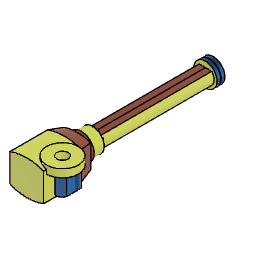
Jaw_3 v3 (Autodesk Fusion 360 design; units mm, degrees)
Autodesk Fusion 360 part; units mm, degrees
sketch "Sketch1" plane through (0, 0, 0) normal (0, 1, 0) x (1, 0, 0)
  line L0 (0, 0) -> (0, 45)
  line L1 (0, 0) -> (0, -45)
  line L2 (0, 45) -> (37.5, 45)
  line L3 (0, 45) -> (-37.5, 45)
  line L4 (0, -45) -> (37.5, -45)
  line L5 (0, -45) -> (-37.5, -45)
  arc A0 (-37.5, 45) -> (-37.5, -45) centre (79.119, 0) ccw
  arc A1 (37.5, -45) -> (37.5, 45) centre (-79.119, 0) ccw
  dimension "d1" = 45
  dimension "d2" = 45
  dimension "d3" = 37.5
  dimension "d4" = 37.5
  dimension "d5" = 37.5
  dimension "d6" = 37.5
  dimension "d7" = 125
  dimension "d8" = 125
  constraint coincident L0.start L1.start
  measures "d1" distance of L0.start L0.end
  measures "d2" distance of L0.start L1.end
  measures "d3" distance of L0.end L2.end
  measures "d4" distance of L0.end L3.end
  measures "d5" distance of L1.end L4.end
  measures "d6" distance of L1.end L5.end
  measures "d7" radius of A0
  measures "d8" radius of A1
sketch "Sketch2" plane through (0, 145, 0) normal (0, 1, 0) x (-1, 0, 0)
  circle A0 centre (0, 0) radius 34.5
  circle A1 centre (0, 0) radius 31
  dimension "d9" = 62
  constraint concentric A0 A1
  measures "d9" diameter of A1
sketch "Sketch3" plane through (0, 135, 0) normal (0, 1, 0) x (-1, 0, 0)
  line L0 (30.8786, 35.6218) -> (-30.8786, 35.6218)
  arc A0 (-30.8786, 35.6218) -> (-30.8786, -35.6218) centre (79.119, 0) ccw
  line L1 (-30.8786, -35.6218) -> (30.8786, -35.6218)
  arc A1 (30.8786, -35.6218) -> (30.8786, 35.6218) centre (-79.119, 0) ccw
  circle A2 centre (0, 0) radius 34.5
  dimension "d10" = 69
  constraint coincident A2.centre origin
  measures "d10" diameter of A2
sketch "Sketch4" plane through (0, 175, 0) normal (0, 1, 0) x (-1, 0, 0)
  circle A0 centre (0, 0) radius 31
  line L0 (0, 0) -> (-27, 0)
  circle A1 centre (-27, 0) radius 2.5
  circle A2 centre (-27, 0) radius 3.5
  dimension "d11" = 27
  dimension "d12" = 5
  dimension "d13" = 1
  constraint coincident A0.centre L0.start
  constraint coincident L0.end A1.centre
  measures "d11" distance of A0.centre L0.end
  measures "d12" diameter of A1
sketch "Sketch5" plane through (0, 175, 0) normal (0, 1, 0) x (-1, 0, 0)
  circle A0 centre (-13.5, 23.3827) radius 3.5
  circle A1 centre (13.5, 23.3827) radius 3.5
  circle A2 centre (27, 0) radius 3.5
  circle A3 centre (13.5, -23.3827) radius 3.5
  circle A4 centre (-13.5, -23.3827) radius 3.5
  circle A5 centre (-27, 0) radius 3.5
  circle A6 centre (0, 0) radius 31
  circle A7 centre (-23.3827, -13.5) radius 3.5
  circle A8 centre (0, -27) radius 3.5
  circle A9 centre (23.3827, -13.5) radius 3.5
  circle A10 centre (23.3827, 13.5) radius 3.5
  circle A11 centre (0, 27) radius 3.5
  circle A12 centre (-23.3827, 13.5) radius 3.5
  line L0 (-15.9819, 0.0787) -> (-15.9461, -16.9213)
  line L1 (-15.9819, 0.0787) -> (-15.9602, 17.0787)
  line L2 (16, 0) -> (16.0134, -16.8465)
  line L3 (16, 0) -> (16, 17)
  arc A13 (-15.9461, -16.9213) -> (16.0134, -16.8465) centre (-0.0069, 0.4409) ccw
  arc A14 (16, 17) -> (-15.9602, 17.0787) centre (-0.0232, -0.4651) ccw
  dimension "d14" = 17
  dimension "d15" = 17
  dimension "d16" = 23.5691
  measures "d14" distance of L0.start L0.end
  measures "d15" distance of L0.start L1.end
  measures "d16" radius of A13
sketch "Sketch6" plane through (0, 275, 0) normal (0, 1, 0) x (-1, 0, 0)
  line L0 (16, 0) -> (16, 17)
  arc A0 (16, 17) -> (-15.9602, 17.0787) centre (-0.0232, -0.4651) ccw
  line L1 (-15.9602, 17.0787) -> (-15.9819, 0.0787)
  line L2 (-15.9819, 0.0787) -> (-15.9461, -16.9213)
  arc A1 (-15.9461, -16.9213) -> (16.0134, -16.8465) centre (-0.0069, 0.4409) ccw
  line L3 (16.0134, -16.8465) -> (16, 0)
  circle A2 centre (0, 0) radius 31
  point P0 (-31, 0)
  constraint coincident A2.centre origin
  constraint coincident A2 P0
sketch "Sketch7" plane through (0, 285, 0) normal (0, 1, 0) x (-1, 0, 0)
  circle A0 centre (0, 0) radius 31
  circle A1 centre (0, 0) radius 30
  dimension "d17" = 1
sketch "Sketch8" plane through (-37.5, 0, -45) normal (-1, 0, 0) x (0, 0, -1)
  circle A0 centre (-90, -50) radius 42.5
  line L0 (-90, 0) -> (-90, -100)
  dimension "d18" = 85
  constraint midpoint A0.centre L0
  measures "d18" diameter of A0
sketch "Sketch9" plane through (0, 286, 0) normal (0, 1, 0) x (-1, 0, 0)
  circle A0 centre (0, 0) radius 30
  circle A1 centre (0, 0) radius 31
  circle A2 centre (0, 0) radius 31
  circle A3 centre (0, 0) radius 31
  constraint coincident A0.centre A1.centre
sketch "Sketch10" plane through (-48, 0, 0) normal (-1, 0, 0) x (0, 0, 1)
  circle A0 centre (45, 50) radius 42.5
  circle A1 centre (45, 50) radius 15
  dimension "d19" = 30
  constraint concentric A0 A1
  measures "d19" diameter of A1
sketch "Sketch11" plane through (0, 70, 0) normal (0, 1, 0) x (-1, 0, 0)
  line L0 (27, 45) -> (27, 75)
  line L1 (27, 75) -> (-8, 75)
  line L2 (-8, 75) -> (-8, 45)
  line L3 (-8, 45) -> (27, 45)
  line L4 (-8, 45) -> (-33, 45)
  line L5 (-8, 45) -> (-8, 87)
  arc A0 (-8, 87) -> (-33, 45) centre (21.8393, 40.7981) ccw
  dimension "d20" = 25
  dimension "d21" = 42
  dimension "d22" = 55
  constraint coincident L2.end L3.start
  measures "d20" distance of L2.end L4.end
  measures "d21" distance of L2.end L5.end
  measures "d22" radius of A0
sketch "Sketch12" plane through (-27, 0, 0) normal (1, 0, 0) x (0, 0, -1)
  line L0 (-45, 7.5) -> (-45, 92.5)
  arc A0 (-45, 92.5) -> (-45, 7.5) centre (-45, 50) ccw
  line L1 (-45, 50) -> (-75, 50)
  line L2 (-45, 70) -> (-75, 70)
  line L3 (-45, 30) -> (-75, 30)
  arc A1 (-75, 70) -> (-75, 30) centre (-52.6393, 50) ccw
  dimension "d23" = 30
  dimension "d24" = 20
  dimension "d25" = 20
  dimension "d26" = 30
  constraint coincident A0.centre L1.start
  measures "d23" distance of A0.centre L1.end
  measures "d26" radius of A1
sketch "Sketch13" plane through (0, 296, 0) normal (0, 1, 0) x (-1, 0, 0)
  circle A0 centre (0, 0) radius 31
  circle A1 centre (0, 0) radius 15
  dimension "d27" = 30
  constraint concentric A0 A1
  measures "d27" diameter of A1
extrude "Extrude1" add sketch "Sketch1" along normal blind 100 makes body 1
extrude "Extrude2" add 1 faces at (15.1807, 100, 3.0661) along direction (0, 1, 0) blind 35 draft -15 on bodies 1 bodies 1
extrude "Extrude3" add sketch "Sketch3" along normal blind 10 contours A2 bodies 1
extrude "Extrude4" add sketch "Sketch2" along normal blind 30 contours A1 bodies 1
extrude "Extrude5" add sketch "Sketch4" along normal blind 2 contours A2 bodies 1
pattern_circular "C-Pattern1" count 12 over 360 about axis through (0, 145, 0) along (0, 1, 0) of "Extrude5"
extrude "Extrude6" add sketch "Sketch5" along normal blind 100 contours L0 L1 L2 L3 A13 A14 bodies 1
extrude "Extrude7" add sketch "Sketch6" along normal blind 10 contours L0 A0 L1 L2 A1 L3 | A2 bodies 1
extrude "Extrude8" add sketch "Sketch7" along normal blind 1 contours A1 bodies 1
extrude "Extrude9" add sketch "Sketch9" along normal blind 10 contours A0 | A1 A2 A3 bodies 1
extrude "Extrude10" add sketch "Sketch8" along normal mid plane 21 bodies 1
extrude "Extrude11" add sketch "Sketch12" along normal blind 35 contours L0 L2 L3 A1 bodies 1
extrude "Extrude12" add sketch "Sketch11" against normal blind 40 contours L2 L4 L5 A0 bodies 1
extrude "Extrude13" cut 1 faces at (8, 50, 85.5464) along direction (1, 0, 0) blind 40 on bodies 1 bodies 1
extrude "Extrude14" cut sketch "Sketch13" against normal blind 20 contours A1 bodies 1
extrude "Extrude15" cut sketch "Sketch10" against normal blind 20 contours A1 bodies 1
move_body "Move1" bodies 1 to x (1, 0, 0) y (0, 1, 0) z (0, 0, 1) at (538.9588, -223.312, 0)
move_body "Move2" bodies 1 to x (-0.866025, 0, 0.5) y (0, 1, 0) z (-0.5, 0, -0.866025) at (-594.2891, 350, 30.5206)
move_body "Align1" bodies 1 to x (-0.5, 0, 0.866025) y (0, 1, 0) z (-0.866025, 0, -0.5) at (-315.713, -176.688, 1040.8886)
ref_plane "WorkPlane1" through (0, 200, 0) normal (0, 1, 0) x (0, 0, 1)
split "Split1" by plane through (0, 200, 0) normal (0, 1, 0) bodies 1 makes body 2 at (-47.2853, 246, -2.5046)
move_body "Move3" bodies 2 to x (1, 0, 0) y (0, 1, 0) z (0, 0, 1) at (0, 200, 0)
loft "Loft1" add section 1 face at (-37.2283, 200, -27.9822) section 2 face at (-37.2283, 400, -27.9822) on bodies 1 2 bodies 1 2
equation "d217 = ( 21 / 2 ) * 1 mm"
